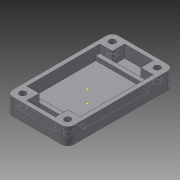
# Autodesk Inventor part: base
Saved by Autodesk Inventor 2015 (Build 190159000, 159)
## iProperties
Created: 2020-03-18
Part Number: base
Material: Generic
Document SubType Name: Modeling
Designer: Toby
Density: 1 g/cm^3
Appearance: Default
Author: Toby
Autodesk Inventor part; units mm, degrees
ref_plane "YZ Plane" through (0, 0, 0) normal (1, 0, 0) x (0, 1, 0)
ref_plane "XZ Plane" through (0, 0, 0) normal (0, 1, 0) x (-1, 0, 0)
ref_plane "XY Plane" through (0, 0, 0) normal (0, 0, 1) x (1, 0, 0)
sketch "Sketch1" plane through (0, 0, 0) normal (0, 0, 1) x (1, 0, 0)
  line L0 (-18.0179, 30.122) -> (11.7821, 30.122)
  line L1 (11.7821, 30.122) -> (11.7821, -21.278)
  line L2 (11.7821, -21.278) -> (-18.0179, -21.278)
  line L3 (-18.0179, -21.278) -> (-18.0179, 30.122)
  point P0 (0, 0)
  dimension "d0" = 29.8
  dimension "d1" = 51.4
  constraints: 8 end point, 2 parallel, 1 horizontal, 1 perpendicular
  measures "d0" distance between parallel lines of L1 L3
  measures "d1" distance between parallel lines of L2 L0
extrude "Extrusion1" add sketch "Sketch1" along normal blind 2
sketch "Sketch2" plane through (0, 0, 2) normal (0, 0, 1) x (1, 0, 0)
  line L0 (-18.0179, 30.122) -> (11.7821, 30.122)
  line L1 (11.7821, 30.122) -> (11.7821, -21.278)
  line L2 (11.7821, -21.278) -> (-18.0179, -21.278)
  line L3 (-18.0179, -21.278) -> (-18.0179, 30.122)
  line L4 (-16.0179, 28.122) -> (9.7821, 28.122)
  line L5 (9.7821, 28.122) -> (9.7821, -19.278)
  line L6 (9.7821, -19.278) -> (-16.0179, -19.278)
  line L7 (-16.0179, -19.278) -> (-16.0179, 28.122)
  point P0 (0, 0)
  dimension "d4" = 2
  dimension "d5" = 2
  dimension "d6" = 2
  dimension "d7" = 2
  dimension "d8" = 25.8
  dimension "d9" = 47.4
  constraints: 16 end point, 4 parallel, 2 horizontal, 2 perpendicular
  measures "d4" distance between parallel lines of L4 L0
  measures "d5" distance between parallel lines of L6 L2
  measures "d6" distance between parallel lines of L3 L7
  measures "d7" distance between parallel lines of L1 L5
  measures "d8" distance between parallel lines of L5 L7
  measures "d9" distance between parallel lines of L6 L4
extrude "Extrusion2" add sketch "Sketch2" along normal blind 6
sketch "Sketch3" plane through (0, 0, 2) normal (0, 0, 1) x (1, 0, 0)
  point P0 (0, 0)
sketch "Sketch4" plane through (0, 0, 2) normal (0, 0, 1) x (1, 0, 0)
  line L0 (-18.0179, 30.122) -> (-10.0179, 30.122)
  line L1 (-10.0179, 30.122) -> (-10.0179, 22.122)
  line L2 (-10.0179, 22.122) -> (-18.0179, 22.122)
  line L3 (-18.0179, 22.122) -> (-18.0179, 30.122)
  line L4 (11.7821, 30.122) -> (3.7821, 30.122)
  line L5 (3.7821, 30.122) -> (3.7821, 22.122)
  line L6 (3.7821, 22.122) -> (11.7821, 22.122)
  line L7 (11.7821, 22.122) -> (11.7821, 30.122)
  line L8 (-18.0179, -21.278) -> (-10.0179, -21.278)
  line L9 (-10.0179, -21.278) -> (-10.0179, -13.278)
  line L10 (-10.0179, -13.278) -> (-18.0179, -13.278)
  line L11 (-18.0179, -13.278) -> (-18.0179, -21.278)
  line L12 (11.7821, -21.278) -> (3.7821, -21.278)
  line L13 (3.7821, -21.278) -> (3.7821, -13.278)
  line L14 (3.7821, -13.278) -> (11.7821, -13.278)
  line L15 (11.7821, -13.278) -> (11.7821, -21.278)
  line L16 (-18.0179, 30.122) -> (-18.0179, -21.278) projected
  line L17 (-18.0179, -21.278) -> (11.7821, -21.278) projected
  point P0 (0, 0)
  dimension "d12" = 8
  dimension "d13" = 8
  dimension "d14" = 8
  dimension "d15" = 8
  dimension "d16" = 8
  dimension "d17" = 8
  dimension "d18" = 8
  dimension "d19" = 8
  dimension "d20" = 35.4
  constraints: 32 end point, 8 parallel, 4 horizontal, 4 perpendicular, 2 collinear
  measures "d12" distance of L1.end L2.end
  measures "d13" distance of L0.end L1.end
  measures "d14" distance of L6.end L5.end
  measures "d15" distance of L5.end L4.end
  measures "d16" distance of L10.end L9.end
  measures "d17" distance of L9.end L8.end
  measures "d18" distance of L13.end L14.end
  measures "d19" distance of L12.end L13.end
  measures "d20" distance between parallel lines of L10 L2
extrude "Extrusion3" add sketch "Sketch4" along normal blind 6
sketch "Sketch5" plane through (0, 0, 2) normal (0, 0, 1) x (1, 0, 0)
  line L0 (9.7821, 22.122) -> (9.7821, -13.278) projected
  line L1 (-16.0179, 22.122) -> (9.7821, 22.122)
  line L2 (9.7821, 22.122) -> (9.7821, 20.122)
  line L3 (9.7821, 20.122) -> (-16.0179, 20.122)
  line L4 (-16.0179, 20.122) -> (-16.0179, 22.122)
  line L5 (-16.0179, -13.278) -> (9.7821, -13.278)
  line L6 (9.7821, -13.278) -> (9.7821, -11.278)
  line L7 (9.7821, -11.278) -> (-16.0179, -11.278)
  line L8 (-16.0179, -11.278) -> (-16.0179, -13.278)
  point P0 (0, 0)
  dimension "d23" = 2
  dimension "d24" = 2
  constraints: 16 end point, 4 parallel, 2 horizontal, 2 perpendicular, 2 point on line
  measures "d23" distance of L1.end L2.end
  measures "d24" distance of L6.end L5.end
extrude "Extrusion4" add sketch "Sketch5" along normal blind 2
sketch "Sketch6" plane through (0, 0, 8) normal (0, 0, 1) x (1, 0, 0)
  point P0 (0, 0)
sketch "Sketch7" plane through (0, 0, 8) normal (0, 0, 1) x (1, 0, 0)
  line L0 (-10.0179, -13.278) -> (-16.0179, -13.278) projected
  line L1 (-18.0179, 30.122) -> (-18.0179, -21.278) projected
  line L2 (9.7821, -13.278) -> (3.7821, -13.278) projected
  line L3 (11.7821, 30.122) -> (11.7821, -21.278) projected
  line L4 (11.7821, 30.122) -> (-18.0179, 30.122) projected
  point P0 (0, 0)
  point P1 (-14.0179, 26.122)
  point P2 (7.7821, 26.122)
  point P3 (-14.0179, -17.278)
  point P4 (7.7821, -17.278)
  dimension "d27" = 4
  dimension "d28" = 4
  dimension "d29" = 4
  dimension "d30" = 4
  dimension "d31" = 4
  dimension "d32" = 4
  dimension "d33" = 4
  dimension "d34" = 4
  measures "d27" distance from line of L0 point (-14.018, -17.278)
  measures "d28" distance from line of L1 point (-14.018, -17.278)
  measures "d29" distance from line of L2 point (7.782, -17.278)
  measures "d30" distance from line of L3 point (7.782, -17.278)
  measures "d31" distance from line of L1 point (-14.018, 26.122)
  measures "d32" distance from line of L4 point (-14.018, 26.122)
  measures "d33" distance from line of L4 point (7.782, 26.122)
  measures "d34" distance from line of L3 point (7.782, 26.122)
hole "Hole1" at (-14.0179, 26.122, 8) at (7.7821, 26.122, 8) at (-14.0179, -17.278, 8) at (7.7821, -17.278, 8) direction (0, 0, -1) diameter 3 depth 6 tip angle 118
fillet "Fillet1" radius 3 4 edges at (-18.0179, -21.278, 4) (11.7821, -21.278, 4) (-18.0179, 30.122, 4) (11.7821, 30.122, 4)
body "Solid1"
